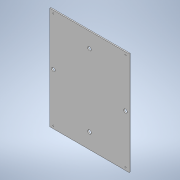
# Autodesk Inventor part: プレート保持_いた
Saved by Autodesk Inventor 2021 (Build 250183000, 183)
## iProperties
Created: 2022-02-09
Part Number: プレート保持_いた
Material: 一般
Document SubType Name: Modeling
Designer: hirohumi
Density: 1 g/cm^3
Appearance: 既定
Author: hirohumi
Autodesk Inventor part; units mm, degrees
ref_plane "YZ Plane" through (0, 0, 0) normal (1, 0, 0) x (0, 1, 0)
ref_plane "XZ Plane" through (0, 0, 0) normal (0, 1, 0) x (-1, 0, 0)
ref_plane "XY Plane" through (0, 0, 0) normal (0, 0, 1) x (1, 0, 0)
sketch "スケッチ1" plane through (0, 0, 0) normal (0, 0, 1) x (1, 0, 0)
  line L0 (0, 100) -> (-100, 0) construction
  line L1 (-100, 0) -> (0, -100) construction
  line L2 (0, -100) -> (100, 0) construction
  line L3 (100, 0) -> (0, 100) construction
  line L4 (0, 100) -> (0, -100) construction
  line L5 (-100, 0) -> (100, 0) construction
  line L6 (100, 135) -> (-100, 135) construction
  line L7 (-100, 135) -> (-100, -135) construction
  line L8 (-100, -135) -> (100, -135) construction
  line L9 (100, -135) -> (100, 135) construction
  line L10 (100, 135) -> (-100, -135) construction
  line L11 (-100, 135) -> (100, -135) construction
  circle A0 centre (-100, 135) radius 1.6
  circle A1 centre (100, 135) radius 1.6
  circle A2 centre (100, -135) radius 1.6
  circle A3 centre (-100, -135) radius 1.6
  circle A4 centre (-100, 0) radius 5
  circle A5 centre (0, 100) radius 5
  circle A6 centre (100, 0) radius 5
  circle A7 centre (0, -100) radius 5
  line L12 (110, 142.5) -> (-110, 142.5)
  line L13 (-110, 142.5) -> (-110, -142.5)
  line L14 (-110, -142.5) -> (110, -142.5)
  line L15 (110, -142.5) -> (110, 142.5)
  line L16 (110, 142.5) -> (-110, -142.5) construction
  line L17 (-110, 142.5) -> (110, -142.5) construction
  point P0 (0, 0)
  point P1 (0, 0)
  dimension "d2" = 200
  dimension "d3" = 270
  dimension "d4" = 3.2
  dimension "d5" = 3.2
  dimension "d6" = 3.2
  dimension "d7" = 3.2
  dimension "d8" = 10
  dimension "d9" = 10
  dimension "d10" = 10
  dimension "d11" = 10
  dimension "d12" = 7.5
  dimension "d19" = 200
  dimension "d20" = 10
  constraints: 34 end point, 8 centre point, 8 coincident, 7 midpoint, 5 parallel, 4 perpendicular, 3 horizontal, 1 vertical alignment, 3 other
  measures "d2" distance of L8.end L7.end
  measures "d3" distance of L7.end L6.end
  measures "d4" diameter of A0
  measures "d5" diameter of A1
  measures "d6" diameter of A2
  measures "d7" diameter of A3
  measures "d8" diameter of A4
  measures "d9" diameter of A5
  measures "d10" diameter of A6
  measures "d11" diameter of A7
  measures "d12" distance from line of L6.end L12
  measures "d19" distance of L0.start L1.end
  measures "d20" distance from line of L13 L0.end
extrude "押し出し1" add sketch "スケッチ1" along normal blind 3
